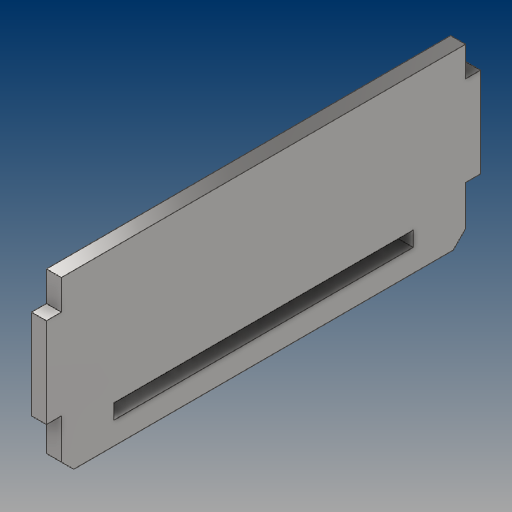
# Autodesk Inventor part: 03_Tam_mat_truoc
Saved by Autodesk Inventor 2021 (Build 250183000, 183)
## iProperties
Created: 2024-04-07
Part Number: 03_Tam_mat_truoc
Material: Stainless Steel, Austenitic
Document SubType Name: Modeling
Designer: Admin
Density: 8 g/cm^3
Appearance: Semi-Polished
Mass: 1944 g
Surface Area: 558 cm^2
Volume: 243 cm^3
Author: Admin
Autodesk Inventor part; units mm, degrees
ref_plane "YZ Plane" through (0, 0, 0) normal (1, 0, 0) x (0, 1, 0)
ref_plane "XZ Plane" through (0, 0, 0) normal (0, 1, 0) x (-1, 0, 0)
ref_plane "XY Plane" through (0, 0, 0) normal (0, 0, 1) x (1, 0, 0)
sketch "Sketch1" plane through (0, 0, 0) normal (1, 0, 0) x (0, 1, 0)
  line L0 (-45, 135) -> (45, 135)
  line L1 (45, 135) -> (45, -135)
  line L2 (45, -135) -> (-45, -135)
  line L3 (-45, -135) -> (-45, 135)
  line L4 (-45, 135) -> (45, -135) construction
  line L5 (45, 135) -> (-45, -135) construction
  point P0 (0, 0)
  dimension "d0" = 90
  dimension "d1" = 270
  constraints: 12 end point, 2 midpoint, 2 parallel, 1 horizontal, 1 perpendicular
  measures "d0" distance of L1.end L2.end
  measures "d1" distance of L0.end L1.end
extrude "Extrusion1" add sketch "Sketch1" along normal blind 10
sketch "Sketch2" plane through (0, 0, 0) normal (-1, 0, 0) x (0, 0, 1)
  line L0 (-135, -45) -> (-135, 45) projected
  line L1 (135, -45) -> (-135, -45) projected
  line L2 (135, 45) -> (135, -45) projected
  line L3 (-135, 45) -> (135, 45) projected
  line L4 (0, 45) -> (0, -5)
  line L5 (145, 25) -> (-145, 25)
  line L6 (-145, 25) -> (-145, -35)
  line L7 (-145, -35) -> (145, -35)
  line L8 (145, -35) -> (145, 25)
  line L9 (145, 25) -> (-145, -35) construction
  line L10 (-145, 25) -> (145, -35) construction
  point P0 (-135, -35)
  point P1 (-135, 25)
  point P2 (135, 25)
  point P3 (135, -35)
  dimension "d8" = 90
  dimension "d9" = 50
  dimension "d10" = 60
  dimension "d11" = 290
  dimension "d12" = 270
  constraints: 14 end point, 3 midpoint, 2 parallel, 1 horizontal, 1 perpendicular, 1 vertical
  measures "d8" distance of L0.start L0.end
  measures "d9" distance of L4.start L4.end
  measures "d10" distance of L5.end L6.end
  measures "d11" distance of L6.end L7.end
  measures "d12" distance of L1.start L0.start
extrude "Extrusion2" add sketch "Sketch2" against normal blind 10 contours L7 L6 L5 L0 | L2 L5 L8 L7
sketch "Sketch3" plane through (10, 0, 0) normal (1, 0, 0) x (0, 0, -1)
  line L0 (135, -45) -> (135, -35) projected
  line L1 (135, -35) -> (145, -35) projected
  line L2 (145, -35) -> (145, 25) projected
  line L3 (145, 25) -> (135, 25) projected
  line L4 (135, 25) -> (135, 45) projected
  line L5 (135, 45) -> (-135, 45) projected
  line L6 (-135, 45) -> (-135, 25) projected
  line L7 (-135, 25) -> (-145, 25) projected
  line L8 (-145, 25) -> (-145, -35) projected
  line L9 (-145, -35) -> (-135, -35) projected
  line L10 (-135, -35) -> (-135, -45) projected
  line L11 (-135, -45) -> (135, -45) projected
  line L12 (135, -20) -> (-135, -20)
  line L13 (-135, -20) -> (-135, -70)
  line L14 (-135, -70) -> (135, -70)
  line L15 (135, -70) -> (135, -20)
  line L16 (135, -20) -> (-135, -70) construction
  line L17 (-135, -20) -> (135, -70) construction
  line L18 (100, -35) -> (-100, -35)
  line L19 (-100, -35) -> (-100, -55)
  line L20 (-100, -55) -> (100, -55)
  line L21 (100, -55) -> (100, -35)
  line L22 (100, -35) -> (-100, -55) construction
  line L23 (-100, -35) -> (100, -55) construction
  point P0 (0, 0)
  point P1 (0, -45)
  point P2 (100, -45)
  point P3 (-100, -45)
  dimension "d13" = 25
  dimension "d14" = 200
  dimension "d15" = 10
  constraints: 24 end point, 5 midpoint, 4 parallel, 2 horizontal, 2 perpendicular, 1 vertical alignment
  measures "d13" distance between parallel lines of L11 L14
  measures "d14" distance between parallel lines of L21 L19
  measures "d15" distance between parallel lines of L11 L20
extrude "Extrusion3" add sketch "Sketch3" against normal blind 10 contours L15 L14 L13 L11 L19 L20 L21
chamfer "Chamfer1" distance 8.25 angle 45 2 edges at (5, -70, 135) (5, -70, -135)
body "Solid1"
